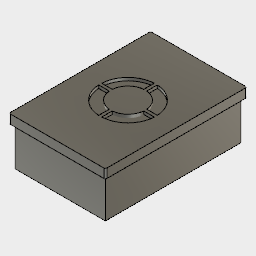
Light_Box_Ver_2.0 (Autodesk Fusion 360 design; units mm, degrees)
Autodesk Fusion 360 part; units mm, degrees
note: some values were not read from the file. Chosen so that the rebuilt part matches the saved one: which bodies a step acts on; which face or edge a step refers to.
sketch "Sketch2" plane through (0, 0, 0) normal (0, 0, 1) x (1, 0, 0)
sketch "Sketch3" plane through (0, 0, 0) normal (0, 0, 1) x (1, 0, 0)
  line L0 (30, 45) -> (-30, 45)
  line L1 (-30, 45) -> (-30, -45)
  line L2 (-30, -45) -> (30, -45)
  line L3 (30, -45) -> (30, 45)
  line L4 (30, 45) -> (-30, -45) construction
  line L5 (-30, 45) -> (30, -45) construction
  circle A0 centre (0, 0) radius 11.5
  circle A1 centre (0, 0) radius 18.5
  line L6 (-10, 1) -> (-19, 1)
  line L7 (-19, 1) -> (-19, -1)
  line L8 (-19, -1) -> (-10, -1)
  line L9 (-10, -1) -> (-10, 1)
  line L10 (1, 11) -> (-1, 11)
  line L11 (-1, 11) -> (-1, 19)
  line L12 (-1, 19) -> (1, 19)
  line L13 (1, 19) -> (1, 11)
  line L14 (10.5, 1) -> (19, 1)
  line L15 (19, 1) -> (19, -1)
  line L16 (19, -1) -> (10.5, -1)
  line L17 (10.5, -1) -> (10.5, 1)
  line L18 (-1, -11) -> (1, -11)
  line L19 (1, -11) -> (1, -19.5)
  line L20 (1, -19.5) -> (-1, -19.5)
  line L21 (-1, -19.5) -> (-1, -11)
  line L22 (29.99, 44.99) -> (-29.99, 44.99)
  line L23 (-29.99, 44.99) -> (-29.99, -44.99)
  line L24 (-29.99, -44.99) -> (29.99, -44.99)
  line L25 (29.99, -44.99) -> (29.99, 44.99)
  line L26 (29.99, 44.99) -> (-29.99, -44.99) construction
  line L27 (-29.99, 44.99) -> (29.99, -44.99) construction
  line L28 (32, 47) -> (-32, 47)
  line L29 (-32, 47) -> (-32, -47)
  line L30 (-32, -47) -> (32, -47)
  line L31 (32, -47) -> (32, 47)
  line L32 (32, 47) -> (-32, -47) construction
  line L33 (-32, 47) -> (32, -47) construction
  dimension "d5" = 60
  dimension "d6" = 90
  dimension "d7" = 23
  dimension "d8" = 37
  dimension "d9" = 89.98
  dimension "d10" = 59.98
  dimension "d13" = 64
  dimension "d14" = 94
  measures "d5" distance of L1.end L2.end
  measures "d6" distance of L0.end L1.end
  measures "d7" diameter of A0
  measures "d8" diameter of A1
  measures "d9" distance of L22.end L23.end
  measures "d10" distance of L23.end L24.end
  measures "d13" distance of L29.end L30.end
  measures "d14" distance of L28.end L29.end
extrude "Extrude2" add sketch "Sketch3" along normal blind 2 contours A1 L14 L15 L16 | A1 L11 L12 L13 | A1 L19 L20 L21 | A1 L6 L7 L8 | L22 L23 L24 L25 makes body 1
extrude "Extrude3" add sketch "Sketch3" along normal blind 2 separate body contours A0 L14 L16 L17 | A0 A1 L14 L16 | A0 L6 L8 L9 L10 L11 L13 L14 L16 L17 L18 L19 L21 | A0 L10 L11 L13 | A0 A1 L11 L13 | A1 L14 L15 L16 | A0 A1 L19 L21 | A0 L18 L19 L21 | A1 L11 L12 L13 | A1 L19 L20 L21 | A0 L6 L8 L9 | A0 A1 L6 L8 | A1 L6 L7 L8 | L22 L23 L24 L25 makes body 2
cylinder "CylinderPrimitive2" add diameter 23 height 7 placed x (0, 1, 0) y (1, 0, 0) z (0, 0, -1) at (0, 0, 0) bodies 2
extrude "Extrude4" add sketch "Sketch3" against normal blind 6 separate body contours L28 L29 L30 L31 makes body 3
fillet "Fillet1" radius 1 4 edges at (-32, 47, -3) (32, 47, -3) (32, -47, -3) (-32, -47, -3) on bodies 3
move_body "Move1" bodies 3 to x (1, 0, 0) y (0, 1, 0) z (0, 0, 1) at (0, 0, 2)
combine "Combine1" operation add target body 1 tool bodies 2 3 makes body 4 at (-31.3333, 15, 2)
box "BoxPrimitive1" add length 89.98 width 59.98 height 30 placed x (0, -1, 0) y (-1, 0, 0) z (0, 0, -1) at (29.99, 44.99, 0) separate body makes body 5
combine "Combine2" operation add target body 1 tool bodies 4 makes body 6 at (-31.3333, 15, 2)
combine "Combine3" operation add target body 1 tool bodies 6 makes body 7 at (-31.3333, 15, 2)
move_face "OffsetFaces1" offset 1 1 faces at (9.9967, 44.99, 0.6667) on bodies 1
move_face "OffsetFaces2" offset 1 1 faces at (-29.99, 15.6633, 0.6667) on bodies 1
move_face "OffsetFaces3" offset 1 1 faces at (-10.6633, -44.99, 1.3333) on bodies 1
move_face "OffsetFaces4" offset 1 1 faces at (29.99, -15.33, 1.3333) on bodies 1
combine "Combine4" operation add target body 1 tool bodies 7
box "BoxPrimitive2" add length 86 width 56 height 5 placed x (0, -1, 0) y (-1, 0, 0) z (0, 0, -1) at (28.01, 42.99, -30) separate body makes body 8
move_face "OffsetFaces5" offset 28 1 faces at (-9.3233, 14.3233, -30) on bodies 8
combine "Combine5" operation cut target body 5 tool bodies 8
